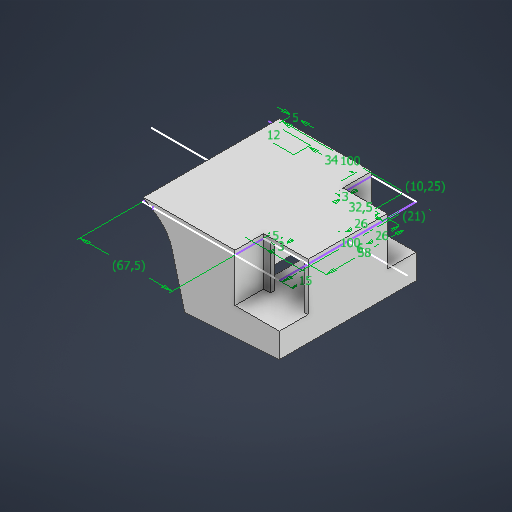
# Autodesk Inventor part: Peçams2
Saved by Autodesk Inventor 2026 (Build 300175050, 175E)
## iProperties
Created: 2025-11-06
Part Number: Peçams2
Material: Genérico
Document SubType Name: Modeling
Designer: luzjl
Density: 1 g/cm^3
Appearance: Padrão
Author: luzjl
Autodesk Inventor part; units mm, degrees
ref_plane "YZ Plane" through (0, 0, 0) normal (1, 0, 0) x (0, 1, 0)
ref_plane "XZ Plane" through (0, 0, 0) normal (0, 1, 0) x (-1, 0, 0)
ref_plane "XY Plane" through (0, 0, 0) normal (0, 0, 1) x (1, 0, 0)
sketch "Esboço1" plane through (0, 0, 0) normal (0, 1, 0) x (-1, 0, 0)
  line L0 (50, 50) -> (-50, 50)
  line L1 (-50, 50) -> (-50, -50)
  line L2 (-50, -50) -> (50, -50)
  line L3 (50, -50) -> (50, 50)
  line L4 (-50, 3) -> (-50, -3)
  line L5 (-50, -3) -> (-50, -29)
  line L6 (-50, -29) -> (-50, -50)
  line L7 (-50, -29) -> (-17.5, -29)
  line L8 (-17.5, -29) -> (-17.5, -50)
  line L9 (-50, -50) -> (-50, 50)
  line L10 (-50, 29) -> (-17.5, 29)
  line L11 (-17.5, 29) -> (-17.5, 50)
  line L12 (24.4193, 35) -> (-9.5807, 35)
  line L13 (-9.5807, 35) -> (-9.5807, -35)
  line L14 (-9.5807, -35) -> (24.4193, -35)
  line L15 (24.4193, -35) -> (24.4193, 35)
  line L16 (-33.75, -29) -> (-39.75, -29)
  line L17 (-39.75, -29) -> (-39.75, -3)
  line L18 (-39.75, -3) -> (-33.75, -3)
  line L19 (-33.75, -3) -> (-27.75, -3)
  line L20 (-27.75, -3) -> (-27.75, -29)
  line L21 (-39.75, 29) -> (-39.75, 3)
  line L22 (-39.75, 3) -> (-33.75, 3)
  line L23 (-33.75, 3) -> (-27.75, 3)
  line L24 (-27.75, 3) -> (-27.75, 29)
  line L25 (50, -50) -> (45, -50)
  line L26 (45, -50) -> (45, 50)
  line L27 (45, 0) -> (42, 0)
  line L28 (-17.5, -29) -> (-14.5, -29)
  line L29 (-14.5, -29) -> (-14.5, -47)
  line L30 (-47, 29) -> (-47, -29)
  line L31 (54.9347, -47) -> (45, -47)
  line L32 (24.4193, -47) -> (-14.5, -47)
  line L33 (-17.5, 29) -> (-14.5, 29)
  line L34 (-14.5, 29) -> (-14.5, 47)
  line L35 (-47, -29) -> (-47, 29)
  line L36 (24.4193, 47) -> (-14.5, 47)
  line L37 (-50, 0) -> (-93.4603, 0)
  line L38 (-76.1073, 0) -> (-50, 0)
  line L39 (-47, 0) -> (56.946, 0)
  line L40 (24.4193, 50) -> (24.4193, -47)
  line L41 (93.4603, 0) -> (45, 0)
  line L42 (24.4193, 0) -> (-47, 0)
  line L43 (24.4193, -47) -> (24.4193, -50)
  line L44 (-17.5, 29) -> (-22.5, 29)
  line L45 (-22.5, 29) -> (-22.5, 26)
  line L46 (-22.5, 26) -> (-14.5, 26)
  line L47 (-14.5, 26) -> (-14.5, 29)
  line L48 (-14.5, -29) -> (-14.5, -26)
  line L49 (-17.5, -29) -> (-22.5, -29)
  line L50 (-22.5, -26) -> (-14.5, -26)
  line L51 (-22.5, -26) -> (-22.5, -29)
  point P0 (0, 0)
  point P1 (7.4193, 0)
  point P2 (42, 50)
  point P3 (-9.5807, 0)
  point P4 (42, -50)
  dimension "d0" = 100
  dimension "d1" = 100
  dimension "d2" = 6
  dimension "d3" = 26
  dimension "d4" = 21
  dimension "d5" = 32.5
  dimension "d6" = 34
  dimension "d10" = 26
  dimension "d12" = 10.25
  dimension "d13" = 67.5
  dimension "d14" = 5
  dimension "d17" = 58
  dimension "d18" = 15
  dimension "d23" = 12
  dimension "d24" = 5
  dimension "d25" = 3
  dimension "d26" = 3
  constraints: 104 end point, 24 point on line, 14 perpendicular, 9 midpoint, 8 horizontal, 5 parallel, 2 collinear, 1 vertical
  measures "d0" distance of L2.end L1.end
  measures "d1" distance of L1.end L0.end
  measures "d2" distance of L4.start L4.end
  measures "d3" distance of L4.end L5.end
  measures "d4" distance of L5.end L1.end
  measures "d5" distance of L5.end L7.end
  measures "d6" distance of L14.end L13.end
  measures "d10" distance of L16.end L17.end
  measures "d12" distance between parallel lines of L5 L17
  measures "d13" distance between parallel lines of L11 L3
  measures "d14" distance of L2.end L25.end
  measures "d17" distance between parallel lines of L7 L10
  measures "d18" distance between parallel lines of L12 L0
  measures "d23" distance between parallel lines of L14 L32
  measures "d24" distance of L11.start L44.end
  measures "d25" distance of L44.end L45.end
  measures "d26" distance of L28.end L48.end
extrude "Extrusão1" add sketch "Esboço1" along normal blind 3 contours L26 L27 L39 L15 L40 L0 | L40 L36 L34 L33 L11 L0 | L26 L2 L43 L40 L15 L39 L27 | L40 L12 L13 L39 L30 L10 L21 L22 L23 L24 L45 L46 L47 L34 L36 | L33 L47 L46 L45 L10 | L15 L39 L13 L12 | L15 L14 L13 L39 | L10 L30 L7 L1 | L2 L8 L28 L29 L32 L43 | L40 L32 L29 L48 L50 L51 L7 L20 L19 L18 L17 L30 L39 L13 L14 | L24 L23 L22 L21 L10 | L7 L51 L50 L48 L28 | L17 L18 L19 L20 L7
extrude "Extrusão2" add sketch "Esboço1" against normal blind 35 contours L40 L36 L34 L33 L11 L0 | L33 L47 L46 L45 L10 | L10 L30 L7 L1 | L2 L8 L28 L29 L32 L43 | L7 L51 L50 L48 L28
sketch "Esboço2" plane through (-45, 3, 50) normal (0, 0, 1) x (1, 0, 0)
  line L0 (0, -3) -> (0, 0) projected
  line L1 (0, -3) -> (13.7317, -11.9575)
  line L2 (0, -3) -> (-4.5989, 0)
  line L3 (-4.5989, 0) -> (0, 0)
  line L4 (20.5807, -3) -> (20.5807, -38) projected
  line L5 (13.7317, -11.9575) -> (20.5807, -38)
  line L6 (0, 0) -> (0, -3)
  line L7 (0, -3) -> (20.5807, -3) projected
  line L8 (0, -3) -> (20.5807, -3)
  line L9 (59.5, -3) -> (20.5807, -3) projected
  line L10 (20.5807, -3) -> (20.5807, -38)
  point P0 (45, -3)
  constraints: 14 end point, 2 perpendicular, 1 collinear, 1 horizontal
extrude "Extrusão3" add sketch "Esboço2" against normal blind 100
sketch "Esboço5" plane through (17.5, -35, 50) normal (0, 0, 1) x (1, 0, 0)
  line L0 (-41.9193, 0) -> (0, 0) projected
  line L1 (-41.9193, 0) -> (-4.8193, 0)
  line L2 (32.5, 0) -> (32.5, 38) projected
  line L3 (-4.8193, 0) -> (32.5, 0)
  line L4 (32.5, 0) -> (32.5, 3)
  line L5 (32.5, 3) -> (-4.8193, 3)
  line L6 (-4.8193, 3) -> (-4.8193, 0)
  point P0 (-17.5, 35)
  dimension "d31" = 37.1
  dimension "d32" = 3
  constraints: 10 end point, 3 perpendicular, 2 point on line
  measures "d31" distance of L0.start L1.end
  measures "d32" distance of L2.start L4.end
extrude "Extrusão4" cut sketch "Esboço5" against normal blind 100.25
extrude "Extrusão5" add sketch "Esboço5" against normal blind 100
sketch "Esboço6" plane through (50, -35, -50) normal (0, 0, -1) x (-1, 0, 0)
  line L0 (37.3193, 0) -> (74.4193, 0) projected
  line L1 (74.4193, 0) -> (81.2683, 26.0425) projected
  line L2 (74.4193, 0) -> (74.4193, -20)
  line L3 (74.4193, 0) -> (0, 0) projected
  line L4 (0, 0) -> (0, -15)
  line L5 (0, -15) -> (74.4193, -20)
  line L6 (74.4193, 0) -> (0, 0)
  point P0 (50, 35)
  dimension "d37" = 20
  dimension "d38" = 15
  constraints: 8 end point, 2 vertical, 1 perpendicular
  measures "d37" distance of L0.end L2.end
  measures "d38" distance of L3.end L4.end
extrude "Extrusão6" add sketch "Esboço6" against normal blind 3
mirror "Espelhar1" about plane through (0, 0, 0) normal (0, 0, 1) of "Extrusão6"
sketch "Esboço7" plane through (0, -35, 0) normal (0, -1, 0) x (1, 0, 0)
  line L0 (50, -50) -> (50, -47) projected
  line L1 (50, -47) -> (47, -47)
  line L2 (-24.4193, -47) -> (50, -47) projected
  line L3 (47, -47) -> (47, 47)
  line L4 (-24.4193, 47) -> (50, 47) projected
  line L5 (47, 47) -> (50, 47)
  line L6 (50, 50) -> (50, 29) projected
  line L7 (50, 47) -> (50, -47)
  point P0 (0, 0)
  dimension "d41" = 3
  constraints: 8 end point, 3 perpendicular, 3 point on line
  measures "d41" distance of L0.end L1.end
extrude "Extrusão7" add sketch "Esboço7" along normal blind 15
sketch "Esboço8" plane through (14.5, 0, 47) normal (0, 0, -1) x (-1, 0, 0)
  line L0 (38.9193, -35) -> (38.9193, -55) projected
  line L1 (38.9193, -35) -> (35.9193, -35)
  line L2 (35.9193, -35) -> (35.9193, -54.7984)
  line L3 (38.9193, -55) -> (-35.5, -50) projected
  line L4 (35.9193, -54.7984) -> (38.9193, -55)
  line L5 (38.9193, -55) -> (38.9193, -35)
  line L6 (45.7683, -8.9575) -> (64.0989, 3) projected
  line L7 (38.9193, -35) -> (45.7683, -8.9575) projected
  line L8 (45.7683, -8.9575) -> (38.9193, -35)
  line L9 (33.7508, -54.6527) -> (44.0879, -15.3473)
  line L10 (33.7508, -54.6527) -> (38.9193, -55)
  line L11 (38.9193, -35) -> (38.9193, -55) projected
  line L12 (38.9193, 0) -> (38.9193, -35) projected
  line L13 (38.9193, -55) -> (38.9193, -35)
  point P0 (14.5, 0)
  dimension "d44" = 3
  constraints: 16 end point, 5 collinear, 2 point on line, 1 horizontal, 1 midpoint, 1 perpendicular
  measures "d44" distance of L0.start L1.end
extrude "Extrusão8" cut sketch "Esboço8" along normal mid plane 260.75 contours L0 L3 L2 L9 | L2 L3 L9
sketch "Esboço9" plane through (14.5, 0, 47) normal (0, 0, -1) x (-1, 0, 0)
  line L0 (33.7508, -54.6527) -> (38.9193, -35) projected
  line L1 (33.7508, -54.6527) -> (30.7576, -54.4516)
  line L2 (33.7508, -54.6527) -> (-35.5, -50) projected
  line L3 (38.9193, -23.6948) -> (30.7576, -54.4516)
  line L4 (38.9193, -35) -> (38.9193, -23.6948)
  line L5 (38.9193, 0) -> (38.9193, -35) projected
  line L6 (38.9193, -35) -> (33.7508, -54.6527)
  line L7 (33.7508, -54.6527) -> (30.7576, -54.4516)
  point P0 (14.5, 0)
  dimension "d47" = 3
  constraints: 10 end point, 2 point on line, 1 collinear
  measures "d47" distance of L0.start L1.end
extrude "Extrusão9" add sketch "Esboço9" along normal blind 95.75
fillet "Arredondamento1" radius 27.75 1 edges at (-31.2683, -8.9575, 0)
